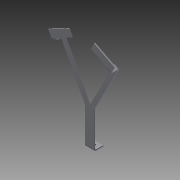
# Autodesk Inventor part: Feeder-Grabber_v2
Saved by Autodesk Inventor 2013 (Build 170138000, 138)
## iProperties
Created: 2013-01-21
Part Number: Feeder-Grabber_v2
Material: Generic
Document SubType Name: Sheet Metal
Designer: motoennies
Density: 1 g/cm^3
Sheet Metal Rule: Default
Author: motoennies
Autodesk Inventor part; units mm, degrees
ref_plane "YZ Plane" through (0, 0, 0) normal (1, 0, 0) x (0, 1, 0)
ref_plane "XZ Plane" through (0, 0, 0) normal (0, 1, 0) x (-1, 0, 0)
ref_plane "XY Plane" through (0, 0, 0) normal (0, 0, 1) x (1, 0, 0)
sketch "Sketch13" plane through (0, 0, 0) normal (0, 0, 1) x (1, 0, 0)
  line L0 (0, 0) -> (25.4, 0)
  line L1 (25.4, 0) -> (25.4, 101.6)
  line L2 (0, 0) -> (0, 101.6)
  line L3 (0, 101.6) -> (-68.9044, 233.9642)
  line L4 (25.4, 101.6) -> (166.7245, 101.6) construction
  line L5 (25.4, 101.6) -> (94.3044, 233.9642)
  line L6 (25.4, 101.6) -> (174.625, 101.6) construction
  line L7 (-68.9044, 233.9642) -> (-57.6394, 239.8284)
  line L8 (12.7, 104.7077) -> (-57.6394, 239.8284)
  line L9 (12.7, 104.7077) -> (-57.6394, 239.8284)
  circle A0 centre (12.7, 123.19) radius 139.7
  line L10 (94.3044, 233.9642) -> (83.0394, 239.8284)
  line L11 (83.0394, 239.8284) -> (12.7, 104.7077)
  dimension "d54" = 25.4
  dimension "d55" = 101.6
  dimension "d56" = 152.5
  dimension "d59" = 149.225
  dimension "d63" = 149.225
  dimension "d64" = 62.5
  dimension "d65" = 12.7
  dimension "d66" = 12.7
  dimension "d82" = 279.4
  dimension "d83" = 123.19
  dimension "d128" = 12.7
  measures "d54" distance of L0.start L0.end
  measures "d55" distance of L0.end L1.end
  measures "d56" angle of L3 L2
  measures "d59" distance of L2.end L3.end
  measures "d63" distance of L1.end L5.end
  measures "d64" angle of L6 L5
  measures "d65" distance of L3.end L7.end
  measures "d66" distance from line of L2 L8.start
  measures "d82" diameter of A0
  measures "d83" distance from line of L0 A0.centre
  measures "d128" distance of L5.end L10.end
extrude "Plate5" add sketch "Sketch13" along normal blind 3.048 contours L2 L3 L7 L8 L11 L10 L5 L1 L0
sketch "Sketch20" plane through (0, 3.048, 3.048) normal (0, -1, 0) x (1, 0, 0)
  line L0 (25.4, 0) -> (0, 0)
  line L1 (0, 0) -> (0, -25.4)
  line L2 (0, -25.4) -> (25.4, -25.4)
  line L3 (25.4, -25.4) -> (25.4, 0)
  constraints: 6 end point, 1 horizontal, 1 perpendicular, 1 vertical
edge flange "Flange7" height 25.4 angle 90 thickness 3.048 bend radius 3.048 thickness toward (0, -1, 0) relief straight relief width 3.048 relief depth 1.524 edges at (12.7, 0, 0) wall of the first edge with corners at (25.4, 3.048, 3.048) (0, 3.048, 3.048) (0, 3.048, -22.352) (25.4, 3.048, -22.352)
bend "Bend7"
corner "Corner7"
sketch "Sketch21" plane through (0, 0, -22.352) normal (0, -1, 0) x (1, 0, 0)
  line L0 (25.4, 0) -> (0, 0) projected
  line L1 (25.4, 19.304) -> (25.4, 0) projected
  circle A0 centre (12.7, 9.652) radius 2.54
  point P0 (0, 22.352)
  dimension "d123" = 5.08
  dimension "d124" = 12.7
  dimension "d125" = 9.652
  constraints: 1 centre point
  measures "d123" diameter of A0
  measures "d124" distance from line of L1 A0.centre
  measures "d125" distance from line of L0 A0.centre
extrude "Cut3" cut sketch "Sketch21" against normal blind 3.048
sketch "Sketch22" plane through (-67.497, 231.2606, 0) normal (-0.4617486, 0.8870108, 0) x (-0.8870108, -0.4617486, 0)
  line L0 (-12.7, 0) -> (0, 0)
  line L1 (0, 0) -> (0, 25.4)
  line L2 (0, 25.4) -> (-12.7, 25.4)
  line L3 (-12.7, 25.4) -> (-12.7, 0)
  constraints: 6 end point, 1 horizontal, 1 perpendicular, 1 vertical
edge flange "Flange8" height 25.4 angle 90 thickness 3.048 bend radius 3.048 thickness toward (-0.4617486, 0.8870108, 0) relief straight relief width 3.048 relief depth 1.524 corner gap 3.048 corner form 0 edges at (-63.2719, 236.8963, 3.048) (88.6719, 236.8963, 3.048) wall of the first edge with corners at (-56.232, 237.1248, 0) (-67.497, 231.2606, 0) (-67.497, 231.2606, 25.4) (-56.232, 237.1248, 25.4)
bend "Bend8"
corner "Corner8"
sketch "Sketch23" plane through (-56.232, 237.1248, 22.352) normal (0, 0, 1) x (1, 0, 0)
  line L0 (-11.265, -5.8642) -> (0, 0)
  line L1 (0, 0) -> (-11.7284, 22.5301)
  line L2 (-11.7284, 22.5301) -> (-22.9935, 16.6659)
  line L3 (-22.9935, 16.6659) -> (-11.265, -5.8642)
  constraints: 6 end point, 1 perpendicular, 2 other
edge flange "Flange9" height 25.4 angle 90 thickness 3.048 bend radius 3.048 thickness toward (0, 0, 1) relief straight relief width 3.048 relief depth 1.524 corner gap 3.048 corner form 0 edges at (-63.2719, 236.8963, 25.4) (88.6719, 236.8963, 25.4) wall of the first edge with corners at (-67.497, 231.2606, 22.352) (-56.232, 237.1248, 22.352) (-67.9604, 259.6549, 22.352) (-79.2254, 253.7907, 22.352)
bend "Bend9"
corner "Corner9"
sketch "Sketch24" plane through (-67.9604, 259.6549, 25.4) normal (0.8870108, 0.4617486, 0) x (0, 0, -1)
  line L0 (0, -19.304) -> (3.048, -19.304) projected
  line L1 (3.048, 0) -> (3.048, -19.304) projected
  line L2 (3.048, 0) -> (0, 0) projected
  line L3 (0, 0) -> (0, -19.304) projected
  point P0 (25.4, -261.6973)
extrude "Extrusion8" add sketch "Sketch24" along normal blind 50.8
sketch "Sketch25" plane through (93.3604, 259.6549, 22.352) normal (-0.8870108, 0.4617486, 0) x (0, 0, 1)
  line L0 (0, -19.304) -> (3.048, -19.304) projected
  line L1 (3.048, -19.304) -> (3.048, 0) projected
  line L2 (0, 0) -> (3.048, 0) projected
  line L3 (0, 0) -> (0, -19.304) projected
  point P0 (-22.352, -273.4257)
extrude "Extrusion9" add sketch "Sketch25" along normal blind 50.8
equation "\"d126\" = Thickness"
equation "\"d113\" = BendReliefWidth"
equation "\"d114\" = BendReliefDepth"
equation "\"d115\" = MinimumRemnant"
equation "\"d116\" = BendRadius"
equation "\"d119\" = BendRadius"
equation "\"d120\" = CornerReliefSize"
equation "\"d121\" = GapSize"
equation "\"d122\" = JacobiRadiusSize"
equation "\"d129\" = BendReliefWidth"
equation "\"d130\" = BendReliefDepth"
equation "\"d131\" = MinimumRemnant"
equation "\"d132\" = BendRadius"
equation "\"d135\" = BendRadius"
equation "\"d136\" = CornerReliefSize"
equation "\"d137\" = GapSize"
equation "\"d138\" = JacobiRadiusSize"
equation "\"d139\" = BendReliefWidth"
equation "\"d140\" = BendReliefDepth"
equation "\"d141\" = MinimumRemnant"
equation "\"d142\" = BendRadius"
equation "\"d145\" = BendRadius"
equation "\"d146\" = CornerReliefSize"
equation "\"d147\" = GapSize"
equation "\"d148\" = JacobiRadiusSize"
equation "\"BendRadius\" = Thickness"
equation "\"BendReliefWidth\" = Thickness"
equation "\"BendReliefDepth\" = 0.5 * Thickness"
equation "\"CornerReliefSize\" = 4 * Thickness"
equation "\"MinimumRemnant\" = 2 * Thickness"
equation "\"TransitionRadius\" = BendRadius"
equation "\"JacobiRadiusSize\" = BendRadius"
equation "\"GapSize\" = Thickness"
equation "\"d2\" = BendRadius"
equation "\"d69\" = BendRadius"
equation "\"Thickness\" = 3.048"
body "Solid3"
